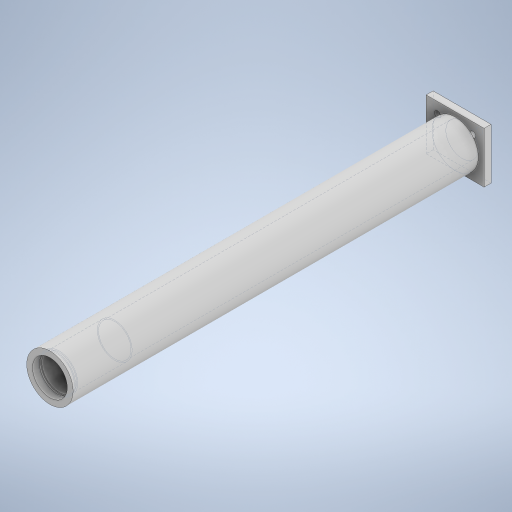
# Autodesk Inventor part: body
Saved by Autodesk Inventor 2023 (Build 270158000, 158)
## iProperties
Created: 2023-07-16
Part Number: body
Material: Generic
Document SubType Name: Modeling
Designer: checo
Density: 1 g/cm^3
Appearance: Default
Author: checo
Autodesk Inventor part; units mm, degrees
ref_plane "YZ Plane" through (0, 0, 0) normal (1, 0, 0) x (0, 1, 0)
ref_plane "XZ Plane" through (0, 0, 0) normal (0, 1, 0) x (-1, 0, 0)
ref_plane "XY Plane" through (0, 0, 0) normal (0, 0, 1) x (1, 0, 0)
sketch "Sketch1" plane through (0, 0, 0) normal (0, 0, 1) x (1, 0, 0)
  circle A0 centre (0, 0) radius 7.5
  circle A1 centre (0, 0) radius 10
  dimension "d0" = 15
  dimension "d1" = 20
  constraints: 2 centre point, 2 coincident
  measures "d0" diameter of A0
  measures "d1" diameter of A1
extrude "Extrusion1" add sketch "Sketch1" along normal blind 24
sketch "Sketch2" plane through (0, 0, 0) normal (0, 0, -1) x (-1, 0, 0)
  circle A0 centre (0, 0) radius 7
  circle A1 centre (0, 0) radius 7.5 projected
  circle A2 centre (0, 0) radius 10 projected
  circle A3 centre (0, 0) radius 7.5 projected
  circle A4 centre (0, 0) radius 10 projected
  circle A5 centre (0, 0) radius 7.5 projected
  circle A6 centre (0, 0) radius 10 projected
  circle A7 centre (0, 0) radius 7.5 projected
  dimension "d4" = 14
  constraints: 1 centre point, 1 coincident
  measures "d4" diameter of A0
extrude "Extrusion2" add sketch "Sketch2" along normal blind 150 contours A1 | A2
sketch "Sketch3" plane through (0, 0, 24) normal (0, 0, 1) x (1, 0, 0)
  circle A0 centre (0, 0) radius 10 projected
  circle A1 centre (0, 0) radius 7.5 projected
  circle A2 centre (0, 0) radius 8
  dimension "d7" = 0.5
  constraints: 1 centre point, 1 coincident
  measures "d7" radial gap between concentric circles of A1 A2
extrude "Extrusion3" add sketch "Sketch3" along normal blind 1 contours A0
sketch "Sketch4" plane through (0, 0, 25) normal (0, 0, 1) x (1, 0, 0)
  circle A0 centre (0, 0) radius 10 projected
  circle A1 centre (0, 0) radius 7.5 projected
extrude "Extrusion4" add sketch "Sketch4" along normal blind 3
sketch "Sketch5" plane through (0, 0, -150) normal (0, 0, -1) x (-1, 0, 0)
  line L0 (-12.5, -10) -> (12.5, -10)
  circle A0 centre (0, 0) radius 10 projected
  line L1 (-12.5, -10) -> (-12.5, 12)
  line L2 (-12.5, 12) -> (12.5, 12)
  line L3 (12.5, 12) -> (12.5, -10)
  circle A1 centre (-7.62, 7.24) radius 1.27
  circle A2 centre (7.62, 7.24) radius 1.27
  line L4 (-7.62, 7.24) -> (7.62, 7.24) construction
  point P0 (0, 7.24)
  point P1 (0, -10)
  point P2 (0, -10)
  point P3 (-7.9828, 6.0229)
  point P4 (-6.423, 7.6645)
  point P5 (6.423, 7.6645)
  point P6 (7.9828, 6.0229)
  dimension "d12" = 25
  dimension "d13" = 22
  dimension "d14" = 15.24
  dimension "d15" = 17.24
  dimension "d16" = 2.54
  constraints: 10 end point, 2 centre point, 2 horizontal, 2 midpoint, 2 vertical, 2 vertical alignment, 1 equal radius, 1 perpendicular, 1 tangent
  measures "d12" distance of L1.end L2.end
  measures "d13" distance of L2.end L0.end
  measures "d14" distance of L4.end L4.start
  measures "d15" distance from line of point (0, 7.24) L0
  measures "d16" diameter of A1
extrude "Extrusion5" add sketch "Sketch5" against normal blind 3
extrude "Extrusion6" cut sketch "Sketch5" against normal blind 3 contours A1 A0 | A0 A1 | A2 A0 | A0 A2
body "Solid1"
